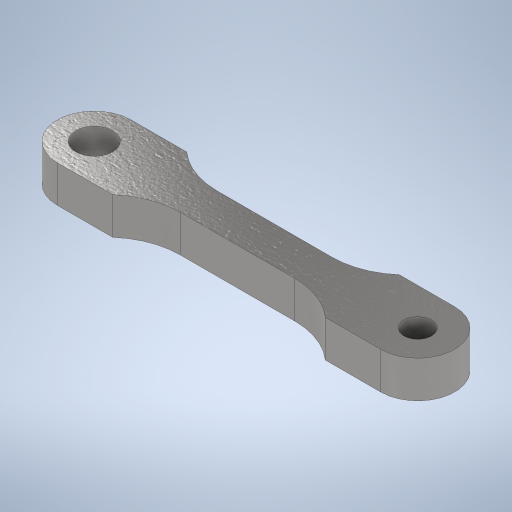
# Autodesk Inventor part: Pleuel
Saved by Autodesk Inventor 2024 (Build 280153000, 153)
## iProperties
Created: 2024-01-15
Part Number: Pleuel
Material: Stahl, galvanisiert
Document SubType Name: Modeling
Designer: ffogue
Density: 7.85 g/cm^3
Appearance: Galvanisiert
Author: ffogue
Autodesk Inventor part; units mm, degrees
ref_plane "YZ Plane" through (0, 0, 0) normal (1, 0, 0) x (0, 1, 0)
ref_plane "XZ Plane" through (0, 0, 0) normal (0, 1, 0) x (-1, 0, 0)
ref_plane "XY Plane" through (0, 0, 0) normal (0, 0, 1) x (1, 0, 0)
sketch "Skizze1" plane through (0, 0, 0) normal (0, 0, 1) x (1, 0, 0)
  line L0 (-21.5, 0) -> (21.5, 0) construction
  line L1 (-11.5, -4) -> (-17.5, -4)
  arc A0 (-17.5, 4) -> (-17.5, -4) centre (-17.5, 0) ccw
  line L2 (-17.5, 4) -> (-11.5, 4)
  line L3 (-6.2085, 2) -> (6.2085, 2)
  line L4 (11.5, 4) -> (17.5, 4)
  arc A1 (17.5, -4) -> (17.5, 4) centre (17.5, 0) ccw
  line L5 (17.5, -4) -> (11.5, -4)
  line L6 (-6.2085, -2) -> (6.2085, -2)
  arc A2 (11.5, -4) -> (6.2085, -2) centre (6.2085, -10) ccw
  arc A3 (-6.2085, -2) -> (-11.5, -4) centre (-6.2085, -10) ccw
  arc A4 (6.2085, 2) -> (11.5, 4) centre (6.2085, 10) ccw
  arc A5 (-11.5, 4) -> (-6.2085, 2) centre (-6.2085, 10) ccw
  point P0 (0, 0)
  point P1 (0, 0)
  dimension "d0" = 8
  dimension "d1" = 8
  dimension "d2" = 4
  dimension "d3" = 6
  dimension "d4" = 6
  dimension "d5" = 35
  dimension "d7" = 8
  constraints: 14 end point, 14 point on circle, 8 tangent, 6 centre point, 5 point on line, 4 parallel, 3 horizontal, 2 equal radius, 1 coincident, 1 midpoint, 1 other
  measures "d0" radius of A3
  measures "d1" radius of A2
  measures "d2" distance between parallel lines of L6 L3
  measures "d3" distance of L4.start L4.end
  measures "d4" distance of L2.start L2.end
  measures "d5" distance of A1.centre A0.centre
  measures "d7" distance between parallel lines of L5 L4
extrude "Extrusion1" add sketch "Skizze1" along normal blind 4
sketch "Skizze2" plane through (0, 0, 4) normal (0, 0, 1) x (1, 0, 0)
  arc A0 (-17.5, 4) -> (-17.5, -4) centre (-17.5, 0) ccw projected
  point P0 (0, 0)
  constraints: 1 coincident
hole "Bohrung1" at (-17.5, 0, 4) direction (0, 0, -1) diameter 4 end through all
sketch "Skizze3" plane through (0, 0, 4) normal (0, 0, 1) x (1, 0, 0)
  arc A0 (17.5, -4) -> (17.5, 4) centre (17.5, 0) ccw projected
  point P0 (0, 0)
  constraints: 1 coincident
hole "Bohrung2" at (17.5, 0, 4) direction (0, 0, -1) diameter 3 end through all
